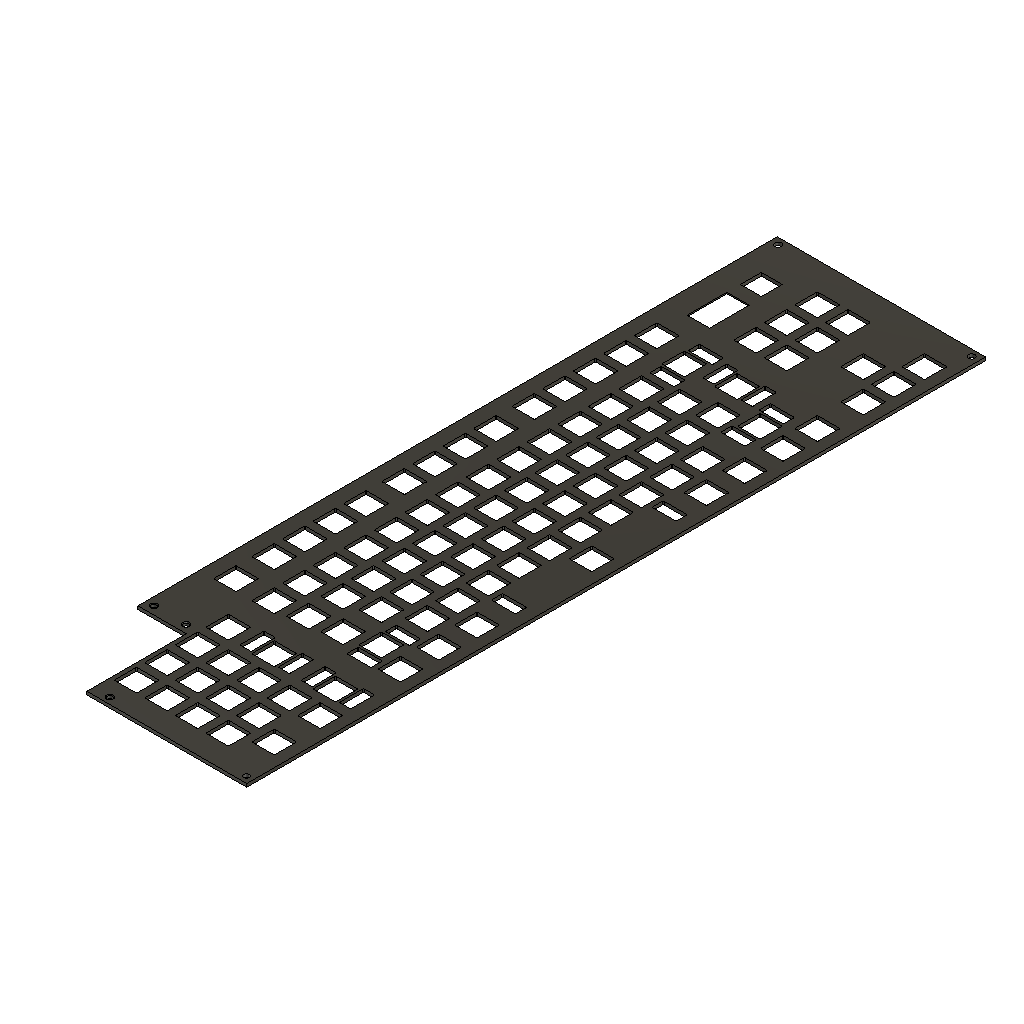
PCBPlate (Autodesk Fusion 360 design; units mm, degrees)
part number: 2026-06-08-16-43-16-633
Autodesk Fusion 360 part; units mm, degrees
(part 1 of 4)
sketch "IronHandPCBPlate" plane through (0, 0, 0) normal (0, 0, 1) x (1, 0, 0)
  arc A0 (-58.5792, -128.4193) -> (-59.0792, -127.9193) centre (-58.5792, -127.9193) cw
  arc A1 (-45.5792, -114.4193) -> (-45.0793, -114.9193) centre (-45.5793, -114.9193) cw
  line L0 (-45.0793, -114.9193) -> (-45.0793, -127.9193)
  line L1 (-59.0792, -127.9193) -> (-59.0793, -114.9193)
  arc A2 (-45.0793, -127.9193) -> (-45.5792, -128.4193) centre (-45.5792, -127.9193) cw
  line L2 (-58.5792, -114.4193) -> (-45.5792, -114.4193)
  line L3 (-45.5792, -128.4193) -> (-58.5792, -128.4193)
  arc A3 (-59.0793, -114.9193) -> (-58.5792, -114.4193) centre (-58.5793, -114.9193) cw
  line L4 (-59.0792, -104.1068) -> (-59.0792, -91.1068)
  line L5 (-45.5792, -104.6068) -> (-58.5792, -104.6068)
  arc A4 (-58.5792, -104.6068) -> (-59.0792, -104.1068) centre (-58.5792, -104.1068) cw
  arc A5 (-45.5793, -90.6068) -> (-45.0792, -91.1068) centre (-45.5792, -91.1068) cw
  arc A6 (-45.0792, -104.1068) -> (-45.5792, -104.6068) centre (-45.5792, -104.1068) cw
  arc A7 (-59.0792, -91.1068) -> (-58.5793, -90.6068) centre (-58.5792, -91.1068) cw
  line L6 (-58.5793, -90.6068) -> (-45.5793, -90.6068)
  line L7 (-45.0792, -91.1068) -> (-45.0792, -104.1068)
  line L8 (-58.5792, -71.5568) -> (-45.5792, -71.5568)
  arc A8 (-45.5792, -71.5568) -> (-45.0792, -72.0568) centre (-45.5792, -72.0568) cw
  line L9 (-45.0792, -72.0568) -> (-45.0792, -85.0568)
  arc A9 (-45.0792, -85.0568) -> (-45.5792, -85.5568) centre (-45.5792, -85.0568) cw
  line L10 (-59.0792, -85.0568) -> (-59.0792, -72.0568)
  line L11 (-45.5792, -85.5568) -> (-58.5792, -85.5568)
  arc A10 (-59.0792, -72.0568) -> (-58.5792, -71.5568) centre (-58.5792, -72.0568) cw
  arc A11 (-58.5792, -85.5568) -> (-59.0792, -85.0568) centre (-58.5792, -85.0568) cw
  arc A12 (-59.0793, -53.0068) -> (-58.5792, -52.5068) centre (-58.5792, -53.0068) cw
  line L12 (-58.5792, -52.5068) -> (-45.5792, -52.5068)
  arc A13 (-58.5792, -66.5068) -> (-59.0792, -66.0068) centre (-58.5792, -66.0068) cw
  line L13 (-45.0792, -53.0068) -> (-45.0793, -66.0068)
  line L14 (-59.0792, -66.0068) -> (-59.0793, -53.0068)
  arc A14 (-45.0793, -66.0068) -> (-45.5792, -66.5068) centre (-45.5792, -66.0068) cw
  arc A15 (-45.5792, -52.5068) -> (-45.0792, -53.0068) centre (-45.5792, -53.0068) cw
  line L15 (-45.5792, -66.5068) -> (-58.5792, -66.5068)
  line L16 (-45.0792, -33.9568) -> (-45.0792, -46.9568)
  line L17 (-58.5792, -33.4568) -> (-45.5792, -33.4568)
  arc A16 (-45.5792, -33.4568) -> (-45.0792, -33.9568) centre (-45.5792, -33.9568) cw
  arc A17 (-45.0792, -46.9568) -> (-45.5792, -47.4568) centre (-45.5792, -46.9568) cw
  arc A18 (-58.5792, -47.4568) -> (-59.0792, -46.9568) centre (-58.5792, -46.9568) cw
  line L18 (-45.5792, -47.4568) -> (-58.5792, -47.4568)
  line L19 (-59.0792, -46.9568) -> (-59.0793, -33.9568)
  arc A19 (-59.0793, -33.9568) -> (-58.5792, -33.4568) centre (-58.5792, -33.9568) cw
  line L20 (-58.5792, -9.6443) -> (-45.5792, -9.6443)
  line L21 (-45.5792, -23.6443) -> (-58.5792, -23.6443)
  arc A20 (-58.5792, -23.6443) -> (-59.0792, -23.1443) centre (-58.5792, -23.1443) cw
  line L22 (-45.0792, -10.1443) -> (-45.0793, -23.1443)
  arc A21 (-59.0793, -10.1443) -> (-58.5792, -9.6443) centre (-58.5792, -10.1443) cw
  arc A22 (-45.0793, -23.1443) -> (-45.5792, -23.6443) centre (-45.5792, -23.1443) cw
  line L23 (-59.0792, -23.1443) -> (-59.0793, -10.1443)
  arc A23 (-45.5792, -9.6443) -> (-45.0792, -10.1443) centre (-45.5792, -10.1443) cw
  line L24 (-45.5792, -4.5943) -> (-58.5792, -4.5943)
  line L25 (-59.0792, -4.0943) -> (-59.0793, 8.9057)
  line L26 (-45.0792, 8.9057) -> (-45.0792, -4.0943)
  arc A24 (-59.0793, 8.9057) -> (-58.5792, 9.4057) centre (-58.5792, 8.9057) cw
  arc A25 (-45.0792, -4.0943) -> (-45.5792, -4.5943) centre (-45.5792, -4.0943) cw
  arc A26 (-58.5792, -4.5943) -> (-59.0792, -4.0943) centre (-58.5792, -4.0943) cw
  line L27 (-58.5792, 9.4057) -> (-45.5792, 9.4057)
  arc A27 (-45.5792, 9.4057) -> (-45.0792, 8.9057) centre (-45.5792, 8.9057) cw
  line L28 (-59.0792, 14.9557) -> (-59.0792, 27.9557)
  line L29 (-45.5792, 14.4557) -> (-58.5792, 14.4557)
  line L30 (-58.5792, 28.4557) -> (-45.5792, 28.4557)
  arc A28 (-45.5792, 28.4557) -> (-45.0792, 27.9557) centre (-45.5792, 27.9557) cw
  arc A29 (-45.0792, 14.9557) -> (-45.5792, 14.4557) centre (-45.5792, 14.9557) cw
  line L31 (-45.0792, 27.9557) -> (-45.0792, 14.9557)
  arc A30 (-59.0792, 27.9557) -> (-58.5792, 28.4557) centre (-58.5792, 27.9557) cw
  arc A31 (-58.5792, 14.4557) -> (-59.0792, 14.9557) centre (-58.5793, 14.9557) cw
  line L32 (-45.5792, 33.5057) -> (-58.5792, 33.5057)
  line L33 (-58.5792, 47.5057) -> (-45.5792, 47.5057)
  line L34 (-45.0792, 47.0057) -> (-45.0792, 34.0057)
  arc A32 (-45.0792, 34.0057) -> (-45.5792, 33.5057) centre (-45.5792, 34.0057) cw
  arc A33 (-58.5792, 33.5057) -> (-59.0792, 34.0057) centre (-58.5792, 34.0057) cw
  line L35 (-59.0792, 34.0057) -> (-59.0793, 47.0057)
  arc A34 (-59.0793, 47.0057) -> (-58.5792, 47.5057) centre (-58.5792, 47.0057) cw
  arc A35 (-45.5792, 47.5057) -> (-45.0792, 47.0057) centre (-45.5792, 47.0057) cw
  arc A36 (-59.0793, 70.8182) -> (-58.5792, 71.3182) centre (-58.5792, 70.8182) cw
  line L36 (-59.0792, 57.8182) -> (-59.0793, 70.8182)
  arc A37 (-45.0792, 57.8182) -> (-45.5792, 57.3182) centre (-45.5792, 57.8182) cw
  line L37 (-45.0792, 70.8182) -> (-45.0792, 57.8182)
  arc A38 (-45.5792, 71.3182) -> (-45.0792, 70.8182) centre (-45.5792, 70.8182) cw
  arc A39 (-58.5792, 57.3182) -> (-59.0792, 57.8182) centre (-58.5792, 57.8182) cw
  line L38 (-45.5792, 57.3182) -> (-58.5792, 57.3182)
  line L39 (-58.5792, 71.3182) -> (-45.5792, 71.3182)
  line L40 (-59.0792, 76.8682) -> (-59.0792, 89.8682)
  arc A40 (-58.5792, 76.3682) -> (-59.0792, 76.8682) centre (-58.5792, 76.8682) cw
  line L41 (-58.5792, 90.3682) -> (-45.5792, 90.3682)
  line L42 (-45.5792, 76.3682) -> (-58.5792, 76.3682)
  arc A41 (-59.0792, 89.8682) -> (-58.5792, 90.3682) centre (-58.5792, 89.8682) cw
  line L43 (-45.0792, 89.8682) -> (-45.0792, 76.8682)
  arc A42 (-45.0792, 76.8682) -> (-45.5792, 76.3682) centre (-45.5792, 76.8682) cw
  arc A43 (-45.5792, 90.3682) -> (-45.0792, 89.8682) centre (-45.5792, 89.8682) cw
  line L44 (-59.0792, 95.9182) -> (-59.0792, 108.9182)
  line L45 (-45.5792, 95.4182) -> (-58.5792, 95.4182)
  arc A44 (-45.0792, 95.9182) -> (-45.5792, 95.4182) centre (-45.5792, 95.9182) cw
  arc A45 (-59.0792, 108.9182) -> (-58.5792, 109.4182) centre (-58.5792, 108.9182) cw
  line L46 (-45.0792, 108.9182) -> (-45.0792, 95.9182)
  arc A46 (-45.5792, 109.4182) -> (-45.0792, 108.9182) centre (-45.5792, 108.9182) cw
  arc A47 (-58.5792, 95.4182) -> (-59.0792, 95.9182) centre (-58.5792, 95.9182) cw
  line L47 (-58.5792, 109.4182) -> (-45.5792, 109.4182)
  line L48 (-58.5792, 128.4682) -> (-45.5792, 128.4682)
  line L49 (-45.5792, 114.4682) -> (-58.5792, 114.4682)
  arc A48 (-59.0792, 127.9682) -> (-58.5792, 128.4682) centre (-58.5792, 127.9682) cw
  line L50 (-45.0792, 127.9682) -> (-45.0792, 114.9682)
  arc A49 (-45.0792, 114.9682) -> (-45.5792, 114.4682) centre (-45.5792, 114.9682) cw
  line L51 (-59.0792, 114.9682) -> (-59.0792, 127.9682)
  arc A50 (-45.5792, 128.4682) -> (-45.0792, 127.9682) centre (-45.5792, 127.9682) cw
  arc A51 (-58.5792, 114.4682) -> (-59.0792, 114.9682) centre (-58.5792, 114.9682) cw
  line L52 (-58.5792, 147.5182) -> (-45.5792, 147.5182)
  line L53 (-59.0792, 134.0182) -> (-59.0793, 147.0182)
  arc A52 (-58.5792, 133.5182) -> (-59.0792, 134.0182) centre (-58.5792, 134.0182) cw
  arc A53 (-45.5792, 147.5182) -> (-45.0792, 147.0182) centre (-45.5792, 147.0182) cw
  line L54 (-45.0792, 147.0182) -> (-45.0792, 134.0182)
  arc A54 (-45.0792, 134.0182) -> (-45.5792, 133.5182) centre (-45.5792, 134.0182) cw
  arc A55 (-59.0793, 147.0182) -> (-58.5792, 147.5182) centre (-58.5792, 147.0182) cw
  line L55 (-45.5792, 133.5182) -> (-58.5792, 133.5182)
  arc A56 (-21.2667, -213.6443) -> (-21.7667, -214.1443) centre (-21.7668, -213.6443) cw
  arc A57 (-21.7667, -200.1443) -> (-21.2668, -200.6443) centre (-21.7667, -200.6443) cw
  line L56 (-21.2668, -200.6443) -> (-21.2667, -213.6443)
  arc A58 (-34.7667, -214.1443) -> (-35.2668, -213.6443) centre (-34.7667, -213.6443) cw
  line L57 (-35.2668, -213.6443) -> (-35.2667, -200.6443)
  line L58 (-21.7667, -214.1443) -> (-34.7667, -214.1443)
  line L59 (-34.7667, -200.1443) -> (-21.7667, -200.1443)
  arc A59 (-35.2667, -200.6443) -> (-34.7667, -200.1443) centre (-34.7667, -200.6443) cw
  line L60 (-34.7667, -181.0943) -> (-21.7667, -181.0943)
  arc A60 (-21.7667, -181.0943) -> (-21.2668, -181.5943) centre (-21.7668, -181.5943) cw
  arc A61 (-21.2667, -194.5943) -> (-21.7668, -195.0943) centre (-21.7667, -194.5943) cw
  arc A62 (-35.2668, -181.5943) -> (-34.7667, -181.0943) centre (-34.7667, -181.5943) cw
  line L61 (-21.2668, -181.5943) -> (-21.2667, -194.5943)
  line L62 (-21.7668, -195.0943) -> (-34.7668, -195.0943)
  arc A63 (-34.7668, -195.0943) -> (-35.2668, -194.5943) centre (-34.7667, -194.5943) cw
  line L63 (-35.2668, -194.5943) -> (-35.2668, -181.5943)
  arc A64 (-21.2667, -175.5443) -> (-21.7667, -176.0443) centre (-21.7667, -175.5443) cw
  arc A65 (-21.7667, -162.0443) -> (-21.2667, -162.5443) centre (-21.7667, -162.5443) cw
  arc A66 (-35.2667, -162.5443) -> (-34.7667, -162.0443) centre (-34.7667, -162.5443) cw
  line L64 (-35.2668, -175.5443) -> (-35.2667, -162.5443)
  line L65 (-34.7667, -162.0443) -> (-21.7667, -162.0443)
  arc A67 (-34.7667, -176.0443) -> (-35.2668, -175.5443) centre (-34.7667, -175.5443) cw
  line L66 (-21.7667, -176.0443) -> (-34.7667, -176.0443)
  line L67 (-21.2667, -162.5443) -> (-21.2667, -175.5443)
  arc A68 (-21.2667, -156.4943) -> (-21.7667, -156.9943) centre (-21.7667, -156.4943) cw
  line L68 (-35.2667, -156.4943) -> (-35.2667, -143.4943)
  line L69 (-21.7667, -156.9943) -> (-34.7667, -156.9943)
  arc A69 (-34.7667, -156.9943) -> (-35.2667, -156.4943) centre (-34.7667, -156.4943) cw
  line L70 (-21.2668, -143.4943) -> (-21.2667, -156.4943)
  arc A70 (-35.2667, -143.4943) -> (-34.7667, -142.9943) centre (-34.7667, -143.4943) cw
  line L71 (-34.7667, -142.9943) -> (-21.7667, -142.9943)
  arc A71 (-21.7667, -142.9943) -> (-21.2668, -143.4943) centre (-21.7667, -143.4943) cw
  arc A72 (-35.2668, -114.9193) -> (-34.7667, -114.4193) centre (-34.7668, -114.9193) cw
  line L72 (-35.2667, -127.9193) -> (-35.2668, -114.9193)
  arc A73 (-21.2667, -127.9193) -> (-21.7667, -128.4193) centre (-21.7667, -127.9193) cw
  arc A74 (-21.7667, -114.4193) -> (-21.2668, -114.9193) centre (-21.7667, -114.9193) cw
  arc A75 (-34.7667, -128.4193) -> (-35.2667, -127.9193) centre (-34.7667, -127.9193) cw
  line L73 (-21.7667, -128.4193) -> (-34.7667, -128.4193)
  line L74 (-34.7667, -114.4193) -> (-21.7667, -114.4193)
  line L75 (-21.2668, -114.9193) -> (-21.2667, -127.9193)
  arc A76 (-35.2667, -95.8693) -> (-34.7667, -95.3693) centre (-34.7667, -95.8693) cw
  arc A77 (-34.7667, -109.3693) -> (-35.2668, -108.8693) centre (-34.7667, -108.8693) cw
  arc A78 (-21.7667, -95.3693) -> (-21.2667, -95.8693) centre (-21.7667, -95.8693) cw
  line L76 (-21.2667, -95.8693) -> (-21.2668, -108.8693)
  arc A79 (-21.2667, -108.8693) -> (-21.7667, -109.3693) centre (-21.7667, -108.8693) cw
  line L77 (-35.2668, -108.8693) -> (-35.2667, -95.8693)
  line L78 (-21.7667, -109.3693) -> (-34.7667, -109.3693)
  line L79 (-34.7667, -95.3693) -> (-21.7667, -95.3693)
  line L80 (-21.7667, -90.3193) -> (-34.7667, -90.3193)
  arc A80 (-34.7667, -90.3193) -> (-35.2667, -89.8193) centre (-34.7667, -89.8193) cw
  line L81 (-21.2667, -76.8193) -> (-21.2667, -89.8193)
  line L82 (-34.7667, -76.3193) -> (-21.7667, -76.3193)
  arc A81 (-21.7667, -76.3193) -> (-21.2667, -76.8193) centre (-21.7667, -76.8193) cw
  line L83 (-35.2667, -89.8193) -> (-35.2667, -76.8193)
  arc A82 (-21.2667, -89.8193) -> (-21.7667, -90.3193) centre (-21.7667, -89.8193) cw
  arc A83 (-35.2667, -76.8193) -> (-34.7667, -76.3193) centre (-34.7667, -76.8193) cw
  line L84 (-21.7667, -71.2693) -> (-34.7667, -71.2693)
  arc A84 (-21.2667, -70.7693) -> (-21.7667, -71.2693) centre (-21.7667, -70.7693) cw
  line L85 (-21.2667, -57.7693) -> (-21.2667, -70.7693)
  arc A85 (-34.7667, -71.2693) -> (-35.2667, -70.7693) centre (-34.7667, -70.7693) cw
  arc A86 (-35.2667, -57.7693) -> (-34.7667, -57.2693) centre (-34.7667, -57.7693) cw
  line L86 (-34.7667, -57.2693) -> (-21.7667, -57.2693)
  line L87 (-35.2667, -70.7693) -> (-35.2667, -57.7693)
  arc A87 (-21.7667, -57.2693) -> (-21.2667, -57.7693) centre (-21.7667, -57.7693) cw
  line L88 (-21.7667, -52.2193) -> (-34.7667, -52.2193)
  line L89 (-34.7667, -38.2193) -> (-21.7667, -38.2193)
  arc A88 (-34.7667, -52.2193) -> (-35.2667, -51.7193) centre (-34.7667, -51.7193) cw
  arc A89 (-21.2667, -51.7193) -> (-21.7667, -52.2193) centre (-21.7667, -51.7193) cw
  line L90 (-21.2667, -38.7193) -> (-21.2667, -51.7193)
  arc A90 (-35.2667, -38.7193) -> (-34.7667, -38.2193) centre (-34.7667, -38.7193) cw
  arc A91 (-21.7667, -38.2193) -> (-21.2667, -38.7193) centre (-21.7667, -38.7193) cw
  line L91 (-35.2667, -51.7193) -> (-35.2667, -38.7193)
  arc A92 (-21.2667, -32.6693) -> (-21.7667, -33.1693) centre (-21.7667, -32.6693) cw
  arc A93 (-21.7667, -19.1693) -> (-21.2667, -19.6693) centre (-21.7667, -19.6693) cw
  line L92 (-34.7667, -19.1693) -> (-21.7667, -19.1693)
  line L93 (-21.2667, -19.6693) -> (-21.2667, -32.6693)
  arc A94 (-34.7667, -33.1693) -> (-35.2667, -32.6693) centre (-34.7667, -32.6693) cw
  line L94 (-21.7667, -33.1693) -> (-34.7667, -33.1693)
  line L95 (-35.2667, -32.6693) -> (-35.2667, -19.6693)
  arc A95 (-35.2667, -19.6693) -> (-34.7667, -19.1693) centre (-34.7667, -19.6693) cw
  arc A96 (-21.2667, -13.6193) -> (-21.7667, -14.1193) centre (-21.7667, -13.6193) cw
  line L96 (-21.2667, -0.6193) -> (-21.2667, -13.6193)
  arc A97 (-34.7667, -14.1193) -> (-35.2667, -13.6193) centre (-34.7667, -13.6193) cw
  line L97 (-35.2667, -13.6193) -> (-35.2667, -0.6193)
  arc A98 (-35.2667, -0.6193) -> (-34.7667, -0.1193) centre (-34.7667, -0.6193) cw
  line L98 (-21.7667, -14.1193) -> (-34.7667, -14.1193)
  arc A99 (-21.7667, -0.1193) -> (-21.2667, -0.6193) centre (-21.7667, -0.6193) cw
  line L99 (-34.7667, -0.1193) -> (-21.7667, -0.1193)
  line L100 (-21.7667, 4.9307) -> (-34.7667, 4.9307)
  arc A100 (-21.7667, 18.9307) -> (-21.2667, 18.4307) centre (-21.7667, 18.4307) cw
  arc A101 (-35.2667, 18.4307) -> (-34.7667, 18.9307) centre (-34.7667, 18.4307) cw
  line L101 (-35.2667, 5.4307) -> (-35.2667, 18.4307)
  line L102 (-21.2667, 18.4307) -> (-21.2667, 5.4307)
  arc A102 (-21.2667, 5.4307) -> (-21.7667, 4.9307) centre (-21.7667, 5.4307) cw
  line L103 (-34.7667, 18.9307) -> (-21.7667, 18.9307)
  arc A103 (-34.7667, 4.9307) -> (-35.2667, 5.4307) centre (-34.7667, 5.4307) cw
  arc A104 (-21.2667, 24.4807) -> (-21.7667, 23.9807) centre (-21.7667, 24.4807) cw
  arc A105 (-21.7667, 37.9807) -> (-21.2667, 37.4807) centre (-21.7667, 37.4807) cw
  arc A106 (-35.2667, 37.4807) -> (-34.7667, 37.9807) centre (-34.7667, 37.4807) cw
  line L104 (-35.2667, 24.4807) -> (-35.2667, 37.4807)
  line L105 (-21.2667, 37.4807) -> (-21.2667, 24.4807)
  arc A107 (-34.7667, 23.9807) -> (-35.2667, 24.4807) centre (-34.7667, 24.4807) cw
  line L106 (-34.7667, 37.9807) -> (-21.7667, 37.9807)
  line L107 (-21.7667, 23.9807) -> (-34.7667, 23.9807)
  line L108 (-21.2667, 56.5307) -> (-21.2667, 43.5307)
  line L109 (-35.2667, 43.5307) -> (-35.2667, 56.5307)
  arc A108 (-35.2667, 56.5307) -> (-34.7667, 57.0307) centre (-34.7667, 56.5307) cw
  line L110 (-34.7667, 57.0307) -> (-21.7667, 57.0307)
  arc A109 (-21.2667, 43.5307) -> (-21.7667, 43.0307) centre (-21.7667, 43.5307) cw
  arc A110 (-21.7667, 57.0307) -> (-21.2667, 56.5307) centre (-21.7667, 56.5307) cw
  line L111 (-21.7667, 43.0307) -> (-34.7667, 43.0307)
  arc A111 (-34.7667, 43.0307) -> (-35.2667, 43.5307) centre (-34.7667, 43.5307) cw
  arc A112 (-21.2667, 62.5807) -> (-21.7667, 62.0807) centre (-21.7667, 62.5807) cw
  line L112 (-34.7667, 76.0807) -> (-21.7667, 76.0807)
  line L113 (-21.7667, 62.0807) -> (-34.7667, 62.0807)
  arc A113 (-35.2667, 75.5807) -> (-34.7667, 76.0807) centre (-34.7667, 75.5807) cw
  arc A114 (-34.7667, 62.0807) -> (-35.2667, 62.5807) centre (-34.7667, 62.5807) cw
  line L114 (-21.2667, 75.5807) -> (-21.2667, 62.5807)
  arc A115 (-21.7667, 76.0807) -> (-21.2667, 75.5807) centre (-21.7667, 75.5807) cw
  line L115 (-35.2667, 62.5807) -> (-35.2667, 75.5807)
  arc A116 (-21.2667, 81.6307) -> (-21.7667, 81.1307) centre (-21.7667, 81.6307) cw
  arc A117 (-34.7667, 81.1307) -> (-35.2667, 81.6307) centre (-34.7667, 81.6307) cw
  line L116 (-34.7667, 95.1307) -> (-21.7667, 95.1307)
  arc A118 (-35.2667, 94.6307) -> (-34.7667, 95.1307) centre (-34.7667, 94.6307) cw
  arc A119 (-21.7667, 95.1307) -> (-21.2667, 94.6307) centre (-21.7667, 94.6307) cw
  line L117 (-21.7667, 81.1307) -> (-34.7667, 81.1307)
  line L118 (-21.2667, 94.6307) -> (-21.2667, 81.6307)
  line L119 (-35.2667, 81.6307) -> (-35.2667, 94.6307)
  line L120 (-35.2667, 100.6807) -> (-35.2667, 113.6807)
  line L121 (-21.2667, 113.6807) -> (-21.2667, 100.6807)
  line L122 (-34.7667, 114.1807) -> (-21.7667, 114.1807)
  line L123 (-21.7667, 100.1807) -> (-34.7667, 100.1807)
  arc A120 (-21.2667, 100.6807) -> (-21.7667, 100.1807) centre (-21.7667, 100.6807) cw
  arc A121 (-21.7667, 114.1807) -> (-21.2667, 113.6807) centre (-21.7667, 113.6807) cw
  arc A122 (-34.7667, 100.1807) -> (-35.2667, 100.6807) centre (-34.7667, 100.6807) cw
  arc A123 (-35.2667, 113.6807) -> (-34.7667, 114.1807) centre (-34.7667, 113.6807) cw
  line L124 (-34.7667, 140.8495) -> (-21.7667, 140.8495)
  line L125 (-21.2667, 140.3495) -> (-21.2667, 127.3495)
  arc A124 (-21.2667, 127.3495) -> (-21.7667, 126.8495) centre (-21.7667, 127.3495) cw
  arc A125 (-34.7667, 126.8495) -> (-35.2667, 127.3495) centre (-34.7667, 127.3495) cw
  line L126 (-35.2667, 127.3495) -> (-35.2667, 140.3495)
  arc A126 (-21.7667, 140.8495) -> (-21.2667, 140.3495) centre (-21.7667, 140.3495) cw
  line L127 (-21.7667, 126.8495) -> (-34.7667, 126.8495)
  arc A127 (-35.2667, 140.3495) -> (-34.7667, 140.8495) centre (-34.7667, 140.3495) cw
  line L128 (-25.7417, 162.5932) -> (-25.7417, 175.5932)
  arc A128 (-12.2417, 176.0932) -> (-11.7417, 175.5932) centre (-12.2417, 175.5932) cw
  line L129 (-25.2417, 176.0932) -> (-12.2417, 176.0932)
  line L130 (-11.7417, 175.5932) -> (-11.7417, 162.5932)
  line L131 (-12.2417, 162.0932) -> (-25.2417, 162.0932)
  arc A129 (-11.7417, 162.5932) -> (-12.2417, 162.0932) centre (-12.2417, 162.5932) cw
  arc A130 (-25.7417, 175.5932) -> (-25.2417, 176.0932) centre (-25.2417, 175.5932) cw
  arc A131 (-25.2417, 162.0932) -> (-25.7417, 162.5932) centre (-25.2417, 162.5932) cw
  arc A132 (-25.7417, 194.6432) -> (-25.2417, 195.1432) centre (-25.2417, 194.6432) cw
  line L132 (-12.2417, 181.1432) -> (-25.2417, 181.1432)
  arc A133 (-11.7417, 181.6432) -> (-12.2417, 181.1432) centre (-12.2417, 181.6432) cw
  line L133 (-11.7417, 194.6432) -> (-11.7417, 181.6432)
  line L134 (-25.2417, 195.1432) -> (-12.2417, 195.1432)
  arc A134 (-25.2417, 181.1432) -> (-25.7417, 181.6432) centre (-25.2417, 181.6432) cw
  line L135 (-25.7417, 181.6432) -> (-25.7417, 194.6432)
  arc A135 (-12.2417, 195.1432) -> (-11.7417, 194.6432) centre (-12.2417, 194.6432) cw
  arc A136 (-11.7417, 200.6932) -> (-12.2417, 200.1932) centre (-12.2417, 200.6932) cw
  line L136 (-25.2417, 214.1932) -> (-12.2417, 214.1932)
  line L137 (-11.7417, 213.6932) -> (-11.7417, 200.6932)
  line L138 (-12.2417, 200.1932) -> (-25.2417, 200.1932)
  arc A137 (-25.7417, 213.6932) -> (-25.2417, 214.1932) centre (-25.2417, 213.6932) cw
  line L139 (-25.7417, 200.6932) -> (-25.7417, 213.6932)
  arc A138 (-25.2417, 200.1932) -> (-25.7417, 200.6932) centre (-25.2417, 200.6932) cw
  arc A139 (-12.2417, 214.1932) -> (-11.7417, 213.6932) centre (-12.2417, 213.6932) cw
  line L140 (-2.7168, -214.1443) -> (-15.7168, -214.1443)
  line L141 (-16.2168, -213.6443) -> (-16.2168, -200.6443)
  arc A140 (-2.2168, -213.6443) -> (-2.7168, -214.1443) centre (-2.7168, -213.6443) cw
  line L142 (-15.7167, -200.1443) -> (-2.7168, -200.1443)
  arc A141 (-2.7168, -200.1443) -> (-2.2167, -200.6443) centre (-2.7167, -200.6443) cw
  line L143 (-2.2167, -200.6443) -> (-2.2168, -213.6443)
  arc A142 (-15.7168, -214.1443) -> (-16.2168, -213.6443) centre (-15.7167, -213.6443) cw
  arc A143 (-16.2168, -200.6443) -> (-15.7167, -200.1443) centre (-15.7168, -200.6443) cw
  arc A144 (-15.7168, -195.0943) -> (-16.2167, -194.5943) centre (-15.7167, -194.5943) cw
  line L144 (-16.2167, -194.5943) -> (-16.2168, -181.5943)
  line L145 (-2.2167, -181.5943) -> (-2.2167, -194.5943)
  line L146 (-15.7167, -181.0943) -> (-2.7168, -181.0943)
  line L147 (-2.7168, -195.0943) -> (-15.7168, -195.0943)
  arc A145 (-2.7168, -181.0943) -> (-2.2168, -181.5943) centre (-2.7167, -181.5943) cw
  arc A146 (-2.2167, -194.5943) -> (-2.7168, -195.0943) centre (-2.7167, -194.5943) cw
  arc A147 (-16.2168, -181.5943) -> (-15.7167, -181.0943) centre (-15.7167, -181.5943) cw
  arc A148 (-2.2168, -175.5443) -> (-2.7168, -176.0443) centre (-2.7167, -175.5443) cw
  arc A149 (-15.7167, -176.0443) -> (-16.2168, -175.5443) centre (-15.7168, -175.5443) cw
  arc A150 (-16.2168, -162.5443) -> (-15.7167, -162.0443) centre (-15.7167, -162.5443) cw
  line L148 (-16.2168, -175.5443) -> (-16.2168, -162.5443)
  arc A151 (-2.7168, -162.0443) -> (-2.2167, -162.5443) centre (-2.7168, -162.5443) cw
  line L149 (-2.2167, -162.5443) -> (-2.2168, -175.5443)
  line L150 (-2.7168, -176.0443) -> (-15.7167, -176.0443)
  line L151 (-15.7167, -162.0443) -> (-2.7168, -162.0443)
  arc A152 (7.3082, -156.4943) -> (6.8083, -156.9943) centre (6.8082, -156.4943) cw
  line L152 (-6.1917, -142.9943) -> (6.8083, -142.9943)
  arc A153 (-6.6917, -143.4943) -> (-6.1917, -142.9943) centre (-6.1917, -143.4943) cw
  line L153 (7.3082, -143.4943) -> (7.3082, -156.4943)
  arc A154 (6.8083, -142.9943) -> (7.3082, -143.4943) centre (6.8083, -143.4943) cw
  line L154 (-6.6917, -156.4943) -> (-6.6917, -143.4943)
  line L155 (6.8083, -156.9943) -> (-6.1917, -156.9943)
  arc A155 (-6.1917, -156.9943) -> (-6.6917, -156.4943) centre (-6.1918, -156.4943) cw
  line L156 (-15.1297, -155.4943) -> (-15.1297, -141.4943)
  arc A156 (-8.6297, -140.9943) -> (-8.1297, -141.4943) centre (-8.6297, -141.4943) cw
  line L157 (-14.6298, -140.9943) -> (-8.6297, -140.9943)
  line L158 (-8.6297, -155.9943) -> (-14.6298, -155.9943)
  arc A157 (-15.1297, -141.4943) -> (-14.6298, -140.9943) centre (-14.6297, -141.4943) cw
  arc A158 (-14.6298, -155.9943) -> (-15.1297, -155.4943) centre (-14.6297, -155.4943) cw
  arc A159 (-8.1297, -155.4943) -> (-8.6297, -155.9943) centre (-8.6297, -155.4943) cw
  line L159 (-8.1297, -141.4943) -> (-8.1297, -155.4943)
  arc A160 (9.2463, -155.9943) -> (8.7463, -155.4943) centre (9.2462, -155.4943) cw
  line L160 (8.7463, -155.4943) -> (8.7463, -141.4943)
  line L161 (15.2463, -155.9943) -> (9.2463, -155.9943)
  line L162 (15.7463, -141.4943) -> (15.7463, -155.4943)
  arc A161 (15.2463, -140.9943) -> (15.7463, -141.4943) centre (15.2463, -141.4943) cw
  arc A162 (8.7463, -141.4943) -> (9.2463, -140.9943) centre (9.2463, -141.4943) cw
  line L163 (9.2463, -140.9943) -> (15.2463, -140.9943)
  arc A163 (15.7463, -155.4943) -> (15.2463, -155.9943) centre (15.2463, -155.4943) cw
  arc A164 (-2.2167, -125.538) -> (-2.7167, -126.038) centre (-2.7167, -125.538) cw
  line L164 (-2.7167, -126.038) -> (-15.7167, -126.038)
  line L165 (-2.2167, -112.538) -> (-2.2167, -125.538)
  line L166 (-15.7167, -112.038) -> (-2.7167, -112.038)
  arc A165 (-2.7167, -112.038) -> (-2.2167, -112.538) centre (-2.7167, -112.538) cw
  line L167 (-16.2168, -125.538) -> (-16.2167, -112.538)
  arc A166 (-16.2167, -112.538) -> (-15.7167, -112.038) centre (-15.7167, -112.538) cw
  arc A167 (-15.7167, -126.038) -> (-16.2168, -125.538) centre (-15.7167, -125.538) cw
  line L168 (-2.2167, -91.1068) -> (-2.2167, -104.1068)
  arc A168 (-2.2167, -104.1068) -> (-2.7167, -104.6068) centre (-2.7167, -104.1068) cw
  line L169 (-16.2167, -104.1068) -> (-16.2167, -91.1068)
  arc A169 (-16.2167, -91.1068) -> (-15.7167, -90.6068) centre (-15.7167, -91.1068) cw
  line L170 (-2.7167, -104.6068) -> (-15.7167, -104.6068)
  arc A170 (-15.7167, -104.6068) -> (-16.2167, -104.1068) centre (-15.7167, -104.1068) cw
  arc A171 (-2.7167, -90.6068) -> (-2.2167, -91.1068) centre (-2.7167, -91.1068) cw
  line L171 (-15.7167, -90.6068) -> (-2.7167, -90.6068)
  line L172 (-2.2167, -72.0568) -> (-2.2167, -85.0568)
  arc A172 (-15.7167, -85.5568) -> (-16.2167, -85.0568) centre (-15.7167, -85.0568) cw
  line L173 (-16.2167, -85.0568) -> (-16.2167, -72.0568)
  arc A173 (-2.7167, -71.5568) -> (-2.2167, -72.0568) centre (-2.7167, -72.0568) cw
  arc A174 (-16.2167, -72.0568) -> (-15.7167, -71.5568) centre (-15.7167, -72.0568) cw
  line L174 (-15.7167, -71.5568) -> (-2.7167, -71.5568)
  arc A175 (-2.2167, -85.0568) -> (-2.7167, -85.5568) centre (-2.7167, -85.0568) cw
  line L175 (-2.7167, -85.5568) -> (-15.7167, -85.5568)
  arc A176 (-15.7167, -66.5068) -> (-16.2167, -66.0068) centre (-15.7167, -66.0068) cw
  line L176 (-2.7167, -66.5068) -> (-15.7167, -66.5068)
  arc A177 (-2.2167, -66.0068) -> (-2.7167, -66.5068) centre (-2.7167, -66.0068) cw
  arc A178 (-2.7167, -52.5068) -> (-2.2167, -53.0068) centre (-2.7167, -53.0068) cw
  line L177 (-2.2167, -53.0068) -> (-2.2167, -66.0068)
  arc A179 (-16.2167, -53.0068) -> (-15.7167, -52.5068) centre (-15.7167, -53.0068) cw
  line L178 (-16.2167, -66.0068) -> (-16.2167, -53.0068)
  line L179 (-15.7167, -52.5068) -> (-2.7167, -52.5068)
  arc A180 (-16.2167, -33.9568) -> (-15.7167, -33.4568) centre (-15.7167, -33.9568) cw
  line L180 (-2.2167, -33.9568) -> (-2.2167, -46.9568)
  line L181 (-16.2167, -46.9568) -> (-16.2167, -33.9568)
  line L182 (-2.7167, -47.4568) -> (-15.7167, -47.4568)
  arc A181 (-2.2167, -46.9568) -> (-2.7167, -47.4568) centre (-2.7167, -46.9568) cw
  arc A182 (-2.7167, -33.4568) -> (-2.2167, -33.9568) centre (-2.7167, -33.9568) cw
  arc A183 (-15.7167, -47.4568) -> (-16.2167, -46.9568) centre (-15.7167, -46.9568) cw
  line L183 (-15.7167, -33.4568) -> (-2.7167, -33.4568)
  arc A184 (-16.2167, -14.9068) -> (-15.7167, -14.4068) centre (-15.7167, -14.9068) cw
  line L184 (-16.2167, -27.9068) -> (-16.2167, -14.9068)
  line L185 (-2.7167, -28.4068) -> (-15.7167, -28.4068)
  arc A185 (-2.2167, -27.9068) -> (-2.7167, -28.4068) centre (-2.7167, -27.9068) cw
  line L186 (-15.7167, -14.4068) -> (-2.7167, -14.4068)
  arc A186 (-15.7167, -28.4068) -> (-16.2167, -27.9068) centre (-15.7167, -27.9068) cw
  line L187 (-2.2167, -14.9068) -> (-2.2167, -27.9068)
  arc A187 (-2.7167, -14.4068) -> (-2.2167, -14.9068) centre (-2.7167, -14.9068) cw
  arc A188 (-16.2167, 4.1432) -> (-15.7167, 4.6432) centre (-15.7167, 4.1432) cw
  line L188 (-2.2167, 4.1432) -> (-2.2167, -8.8568)
  line L189 (-2.7167, -9.3568) -> (-15.7167, -9.3568)
  line L190 (-16.2167, -8.8568) -> (-16.2167, 4.1432)
  arc A189 (-2.7167, 4.6432) -> (-2.2167, 4.1432) centre (-2.7167, 4.1432) cw
  arc A190 (-2.2167, -8.8568) -> (-2.7167, -9.3568) centre (-2.7167, -8.8568) cw
  arc A191 (-15.7167, -9.3568) -> (-16.2167, -8.8568) centre (-15.7167, -8.8568) cw
  line L191 (-15.7167, 4.6432) -> (-2.7167, 4.6432)
  arc A192 (-2.7167, 23.6932) -> (-2.2167, 23.1932) centre (-2.7167, 23.1932) cw
  arc A193 (-15.7167, 9.6932) -> (-16.2167, 10.1932) centre (-15.7167, 10.1932) cw
  line L192 (-2.2167, 23.1932) -> (-2.2167, 10.1932)
  line L193 (-16.2167, 10.1932) -> (-16.2167, 23.1932)
  arc A194 (-2.2167, 10.1932) -> (-2.7167, 9.6932) centre (-2.7167, 10.1932) cw
  arc A195 (-16.2167, 23.1932) -> (-15.7167, 23.6932) centre (-15.7167, 23.1932) cw
  line L194 (-15.7167, 23.6932) -> (-2.7167, 23.6932)
  line L195 (-2.7167, 9.6932) -> (-15.7167, 9.6932)
  arc A196 (-2.7167, 42.7432) -> (-2.2167, 42.2432) centre (-2.7167, 42.2432) cw
  line L196 (-2.7167, 28.7432) -> (-15.7167, 28.7432)
  line L197 (-15.7167, 42.7432) -> (-2.7167, 42.7432)
  line L198 (-2.2167, 42.2432) -> (-2.2167, 29.2432)
  arc A197 (-2.2167, 29.2432) -> (-2.7167, 28.7432) centre (-2.7167, 29.2432) cw
  arc A198 (-15.7167, 28.7432) -> (-16.2167, 29.2432) centre (-15.7167, 29.2432) cw
  line L199 (-16.2167, 29.2432) -> (-16.2167, 42.2432)
  arc A199 (-16.2167, 42.2432) -> (-15.7167, 42.7432) centre (-15.7167, 42.2432) cw
  line L200 (-16.2167, 48.2932) -> (-16.2167, 61.2932)
  line L201 (-2.7167, 47.7932) -> (-15.7167, 47.7932)
  arc A200 (-2.7167, 61.7932) -> (-2.2167, 61.2932) centre (-2.7167, 61.2932) cw
  line L202 (-2.2167, 61.2932) -> (-2.2167, 48.2932)
  arc A201 (-16.2167, 61.2932) -> (-15.7167, 61.7932) centre (-15.7167, 61.2932) cw
  arc A202 (-2.2167, 48.2932) -> (-2.7167, 47.7932) centre (-2.7167, 48.2932) cw
  arc A203 (-15.7167, 47.7932) -> (-16.2167, 48.2932) centre (-15.7167, 48.2932) cw
  line L203 (-15.7167, 61.7932) -> (-2.7167, 61.7932)
  arc A204 (-2.7167, 80.8432) -> (-2.2167, 80.3432) centre (-2.7167, 80.3432) cw
  line L204 (-16.2167, 67.3432) -> (-16.2167, 80.3432)
  line L205 (-2.2167, 80.3432) -> (-2.2167, 67.3432)
  arc A205 (-15.7167, 66.8432) -> (-16.2167, 67.3432) centre (-15.7167, 67.3432) cw
  line L206 (-2.7167, 66.8432) -> (-15.7167, 66.8432)
  line L207 (-15.7167, 80.8432) -> (-2.7167, 80.8432)
  arc A206 (-16.2167, 80.3432) -> (-15.7167, 80.8432) centre (-15.7167, 80.3432) cw
  arc A207 (-2.2167, 67.3432) -> (-2.7167, 66.8432) centre (-2.7167, 67.3432) cw
  line L208 (-15.7167, 99.8932) -> (-2.7167, 99.8932)
  arc A208 (-2.7167, 99.8932) -> (-2.2167, 99.3932) centre (-2.7167, 99.3932) cw
  arc A209 (-16.2167, 99.3932) -> (-15.7167, 99.8932) centre (-15.7167, 99.3932) cw
  arc A210 (-2.2167, 86.3932) -> (-2.7167, 85.8932) centre (-2.7167, 86.3932) cw
  line L209 (-2.7167, 85.8932) -> (-15.7167, 85.8932)
  line L210 (-2.2167, 99.3932) -> (-2.2167, 86.3932)
  line L211 (-16.2167, 86.3932) -> (-16.2167, 99.3932)
  arc A211 (-15.7167, 85.8932) -> (-16.2167, 86.3932) centre (-15.7167, 86.3932) cw
  line L212 (-16.2167, 105.4432) -> (-16.2167, 118.4432)
  arc A212 (-16.2167, 118.4432) -> (-15.7167, 118.9432) centre (-15.7167, 118.4432) cw
  arc A213 (-15.7167, 104.9432) -> (-16.2167, 105.4432) centre (-15.7167, 105.4432) cw
  line L213 (-2.7167, 104.9432) -> (-15.7167, 104.9432)
  arc A214 (-2.2167, 105.4432) -> (-2.7167, 104.9432) centre (-2.7167, 105.4432) cw
  arc A215 (-2.7167, 118.9432) -> (-2.2167, 118.4432) centre (-2.7167, 118.4432) cw
  line L214 (-2.2167, 118.4432) -> (-2.2167, 105.4432)
  line L215 (-15.7167, 118.9432) -> (-2.7167, 118.9432)
  line L216 (6.8083, 131.137) -> (-6.1917, 131.137)
  arc A216 (-6.6917, 144.637) -> (-6.1917, 145.137) centre (-6.1917, 144.637) cw
  arc A217 (6.8083, 145.137) -> (7.3083, 144.637) centre (6.8083, 144.637) cw
  line L217 (7.3083, 144.637) -> (7.3083, 131.637)
  arc A218 (-6.1917, 131.137) -> (-6.6917, 131.637) centre (-6.1917, 131.637) cw
  line L218 (-6.1917, 145.137) -> (6.8083, 145.137)
  arc A219 (7.3083, 131.637) -> (6.8083, 131.137) centre (6.8083, 131.637) cw
  line L219 (-6.6917, 131.637) -> (-6.6917, 144.637)
  arc A220 (-8.6297, 147.137) -> (-8.1297, 146.637) centre (-8.6297, 146.637) cw
  line L220 (-14.6297, 147.137) -> (-8.6297, 147.137)
  arc A221 (-14.6297, 132.137) -> (-15.1297, 132.637) centre (-14.6297, 132.637) cw
  line L221 (-15.1297, 132.637) -> (-15.1297, 146.637)
  arc A222 (-8.1297, 132.637) -> (-8.6297, 132.137) centre (-8.6297, 132.637) cw
  line L222 (-8.6297, 132.137) -> (-14.6297, 132.137)
  arc A223 (-15.1297, 146.637) -> (-14.6297, 147.137) centre (-14.6297, 146.637) cw
  line L223 (-8.1297, 146.637) -> (-8.1297, 132.637)
  line L224 (15.2463, 132.137) -> (9.2463, 132.137)
  line L225 (15.7463, 146.637) -> (15.7463, 132.637)
  line L226 (8.7463, 132.637) -> (8.7463, 146.637)
  arc A224 (9.2463, 132.137) -> (8.7463, 132.637) centre (9.2463, 132.637) cw
  arc A225 (15.7463, 132.637) -> (15.2463, 132.137) centre (15.2463, 132.637) cw
  arc A226 (8.7463, 146.637) -> (9.2463, 147.137) centre (9.2463, 146.637) cw
  arc A227 (15.2463, 147.137) -> (15.7463, 146.637) centre (15.2463, 146.637) cw
  line L227 (9.2463, 147.137) -> (15.2463, 147.137)
  line L228 (-6.1917, 176.0932) -> (6.8083, 176.0932)
  arc A228 (-6.1917, 162.0932) -> (-6.6917, 162.5932) centre (-6.1917, 162.5932) cw
  line L229 (6.8083, 162.0932) -> (-6.1917, 162.0932)
  arc A229 (-6.6917, 175.5932) -> (-6.1917, 176.0932) centre (-6.1917, 175.5932) cw
  line L230 (7.3083, 175.5932) -> (7.3083, 162.5932)
  arc A230 (6.8083, 176.0932) -> (7.3083, 175.5932) centre (6.8083, 175.5932) cw
  arc A231 (7.3083, 162.5932) -> (6.8083, 162.0932) centre (6.8083, 162.5932) cw
  line L231 (-6.6917, 162.5932) -> (-6.6917, 175.5932)
  arc A232 (-6.6917, 194.6432) -> (-6.1917, 195.1432) centre (-6.1917, 194.6432) cw
  line L232 (7.3083, 194.6432) -> (7.3083, 181.6432)
  arc A233 (7.3083, 181.6432) -> (6.8083, 181.1432) centre (6.8083, 181.6432) cw
  arc A234 (-6.1917, 181.1432) -> (-6.6917, 181.6432) centre (-6.1917, 181.6432) cw
  line L233 (-6.6917, 181.6432) -> (-6.6917, 194.6432)
  line L234 (6.8083, 181.1432) -> (-6.1917, 181.1432)
  arc A235 (6.8083, 195.1432) -> (7.3083, 194.6432) centre (6.8083, 194.6432) cw
  line L235 (-6.1917, 195.1432) -> (6.8083, 195.1432)
  arc A236 (6.8083, 214.1932) -> (7.3083, 213.6932) centre (6.8083, 213.6932) cw
  arc A237 (-6.6917, 213.6932) -> (-6.1917, 214.1932) centre (-6.1917, 213.6932) cw
  line L236 (-6.1917, 214.1932) -> (6.8083, 214.1932)
  line L237 (-6.6917, 200.6932) -> (-6.6917, 213.6932)
  line L238 (7.3083, 213.6932) -> (7.3083, 200.6932)
  line L239 (6.8083, 200.1932) -> (-6.1917, 200.1932)
  arc A238 (7.3083, 200.6932) -> (6.8083, 200.1932) centre (6.8083, 200.6932) cw
  arc A239 (-6.1917, 200.1932) -> (-6.6917, 200.6932) centre (-6.1917, 200.6932) cw
  line L240 (16.8333, -200.6443) -> (16.8332, -213.6443)
  arc A240 (2.8332, -200.6443) -> (3.3332, -200.1443) centre (3.3332, -200.6443) cw
  arc A241 (16.8332, -213.6443) -> (16.3333, -214.1443) centre (16.3332, -213.6443) cw
  line L241 (16.3333, -214.1443) -> (3.3332, -214.1443)
  arc A242 (3.3332, -214.1443) -> (2.8332, -213.6443) centre (3.3333, -213.6443) cw
  arc A243 (16.3333, -200.1443) -> (16.8333, -200.6443) centre (16.3333, -200.6443) cw
  line L242 (2.8332, -213.6443) -> (2.8332, -200.6443)
  line L243 (3.3332, -200.1443) -> (16.3333, -200.1443)
  arc A244 (3.3332, -195.0943) -> (2.8333, -194.5943) centre (3.3332, -194.5943) cw
  arc A245 (16.3333, -181.0943) -> (16.8333, -181.5943) centre (16.3333, -181.5943) cw
  line L244 (3.3332, -181.0943) -> (16.3333, -181.0943)
  line L245 (2.8333, -194.5943) -> (2.8332, -181.5943)
  arc A246 (16.8333, -194.5943) -> (16.3333, -195.0943) centre (16.3333, -194.5943) cw
  line L246 (16.3333, -195.0943) -> (3.3332, -195.0943)
  arc A247 (2.8332, -181.5943) -> (3.3332, -181.0943) centre (3.3333, -181.5943) cw
  line L247 (16.8333, -181.5943) -> (16.8333, -194.5943)
  arc A248 (16.8332, -175.5443) -> (16.3333, -176.0443) centre (16.3333, -175.5443) cw
  arc A249 (2.8332, -162.5443) -> (3.3332, -162.0443) centre (3.3333, -162.5443) cw
  line L248 (16.8333, -162.5443) -> (16.8332, -175.5443)
  line L249 (16.3333, -176.0443) -> (3.3332, -176.0443)
  line L250 (3.3332, -162.0443) -> (16.3333, -162.0443)
  arc A250 (16.3333, -162.0443) -> (16.8333, -162.5443) centre (16.3333, -162.5443) cw
  arc A251 (3.3332, -176.0443) -> (2.8333, -175.5443) centre (3.3332, -175.5443) cw
  line L251 (2.8333, -175.5443) -> (2.8332, -162.5443)
  line L252 (16.8333, -110.1568) -> (16.8333, -123.1568)
  line L253 (3.3333, -109.6568) -> (16.3333, -109.6568)
  arc A252 (3.3333, -123.6568) -> (2.8333, -123.1568) centre (3.3333, -123.1568) cw
  arc A253 (16.3333, -109.6568) -> (16.8333, -110.1568) centre (16.3333, -110.1568) cw
  arc A254 (16.8333, -123.1568) -> (16.3333, -123.6568) centre (16.3333, -123.1568) cw
  line L254 (16.3333, -123.6568) -> (3.3333, -123.6568)
  arc A255 (2.8333, -110.1568) -> (3.3333, -109.6568) centre (3.3333, -110.1568) cw
  line L255 (2.8333, -123.1568) -> (2.8333, -110.1568)
  line L256 (16.8333, -86.3443) -> (16.8333, -99.3443)
  arc A256 (3.3333, -99.8443) -> (2.8333, -99.3443) centre (3.3333, -99.3443) cw
  line L257 (16.3333, -99.8443) -> (3.3333, -99.8443)
  line L258 (3.3333, -85.8443) -> (16.3333, -85.8443)
  line L259 (2.8333, -99.3443) -> (2.8332, -86.3443)
  arc A257 (2.8332, -86.3443) -> (3.3333, -85.8443) centre (3.3333, -86.3443) cw
  arc A258 (16.8333, -99.3443) -> (16.3333, -99.8443) centre (16.3333, -99.3443) cw
  arc A259 (16.3333, -85.8443) -> (16.8333, -86.3443) centre (16.3333, -86.3443) cw
  arc A260 (16.8333, -80.2943) -> (16.3333, -80.7943) centre (16.3333, -80.2943) cw
  line L260 (16.3333, -80.7943) -> (3.3333, -80.7943)
  line L261 (2.8333, -80.2943) -> (2.8333, -67.2943)
  line L262 (3.3333, -66.7943) -> (16.3333, -66.7943)
  arc A261 (16.3333, -66.7943) -> (16.8333, -67.2943) centre (16.3333, -67.2943) cw
  arc A262 (3.3333, -80.7943) -> (2.8333, -80.2943) centre (3.3333, -80.2943) cw
  line L263 (16.8333, -67.2943) -> (16.8333, -80.2943)
  arc A263 (2.8333, -67.2943) -> (3.3333, -66.7943) centre (3.3333, -67.2943) cw
  line L264 (3.3333, -47.7443) -> (16.3333, -47.7443)
  arc A264 (16.8333, -61.2443) -> (16.3333, -61.7443) centre (16.3333, -61.2443) cw
  line L265 (2.8333, -61.2443) -> (2.8333, -48.2443)
  line L266 (16.3333, -61.7443) -> (3.3333, -61.7443)
  arc A265 (2.8333, -48.2443) -> (3.3333, -47.7443) centre (3.3333, -48.2443) cw
  line L267 (16.8333, -48.2443) -> (16.8333, -61.2443)
  arc A266 (3.3333, -61.7443) -> (2.8333, -61.2443) centre (3.3333, -61.2443) cw
  arc A267 (16.3333, -47.7443) -> (16.8333, -48.2443) centre (16.3333, -48.2443) cw
  line L268 (3.3333, -28.6943) -> (16.3333, -28.6943)
  arc A268 (16.8333, -42.1943) -> (16.3333, -42.6943) centre (16.3333, -42.1943) cw
  arc A269 (3.3333, -42.6943) -> (2.8333, -42.1943) centre (3.3333, -42.1943) cw
  arc A270 (2.8333, -29.1943) -> (3.3333, -28.6943) centre (3.3333, -29.1943) cw
  line L269 (2.8333, -42.1943) -> (2.8333, -29.1943)
  arc A271 (16.3333, -28.6943) -> (16.8333, -29.1943) centre (16.3333, -29.1943) cw
  line L270 (16.3333, -42.6943) -> (3.3333, -42.6943)
  line L271 (16.8333, -29.1943) -> (16.8333, -42.1943)
  line L272 (16.8333, -10.1443) -> (16.8333, -23.1443)
  arc A272 (3.3333, -23.6443) -> (2.8333, -23.1443) centre (3.3333, -23.1443) cw
  line L273 (2.8333, -23.1443) -> (2.8333, -10.1443)
  line L274 (3.3333, -9.6443) -> (16.3333, -9.6443)
  line L275 (16.3333, -23.6443) -> (3.3333, -23.6443)
  arc A273 (16.3333, -9.6443) -> (16.8333, -10.1443) centre (16.3333, -10.1443) cw
  arc A274 (2.8333, -10.1443) -> (3.3333, -9.6443) centre (3.3333, -10.1443) cw
  arc A275 (16.8333, -23.1443) -> (16.3333, -23.6443) centre (16.3333, -23.1443) cw
  line L276 (16.8333, 8.9057) -> (16.8333, -4.0943)
  line L277 (16.3333, -4.5943) -> (3.3333, -4.5943)
  arc A276 (16.8333, -4.0943) -> (16.3333, -4.5943) centre (16.3333, -4.0943) cw
  arc A277 (3.3333, -4.5943) -> (2.8333, -4.0943) centre (3.3333, -4.0943) cw
  arc A278 (16.3333, 9.4057) -> (16.8333, 8.9057) centre (16.3333, 8.9057) cw
  line L278 (2.8333, -4.0943) -> (2.8333, 8.9057)
  line L279 (3.3333, 9.4057) -> (16.3333, 9.4057)
  arc A279 (2.8333, 8.9057) -> (3.3333, 9.4057) centre (3.3333, 8.9057) cw
  arc A280 (2.8333, 27.9557) -> (3.3333, 28.4557) centre (3.3333, 27.9557) cw
  arc A281 (16.8333, 14.9557) -> (16.3333, 14.4557) centre (16.3333, 14.9557) cw
  arc A282 (3.3333, 14.4557) -> (2.8333, 14.9557) centre (3.3333, 14.9557) cw
  arc A283 (16.3333, 28.4557) -> (16.8333, 27.9557) centre (16.3333, 27.9557) cw
  line L280 (16.3333, 14.4557) -> (3.3333, 14.4557)
  line L281 (16.8333, 27.9557) -> (16.8333, 14.9557)
  line L282 (3.3333, 28.4557) -> (16.3333, 28.4557)
  line L283 (2.8333, 14.9557) -> (2.8333, 27.9557)
  arc A284 (16.3333, 47.5057) -> (16.8333, 47.0057) centre (16.3333, 47.0057) cw
  line L284 (2.8333, 34.0057) -> (2.8333, 47.0057)
  line L285 (3.3333, 47.5057) -> (16.3333, 47.5057)
  arc A285 (16.8333, 34.0057) -> (16.3333, 33.5057) centre (16.3333, 34.0057) cw
  line L286 (16.8333, 47.0057) -> (16.8333, 34.0057)
  line L287 (16.3333, 33.5057) -> (3.3333, 33.5057)
  arc A286 (2.8333, 47.0057) -> (3.3333, 47.5057) centre (3.3333, 47.0057) cw
  arc A287 (3.3333, 33.5057) -> (2.8333, 34.0057) centre (3.3333, 34.0057) cw
  line L288 (16.3333, 52.5557) -> (3.3333, 52.5557)
  arc A288 (16.8333, 53.0557) -> (16.3333, 52.5557) centre (16.3333, 53.0557) cw
  line L289 (2.8333, 53.0557) -> (2.8333, 66.0557)
  arc A289 (3.3333, 52.5557) -> (2.8333, 53.0557) centre (3.3333, 53.0557) cw
  line L290 (3.3333, 66.5557) -> (16.3333, 66.5557)
  line L291 (16.8333, 66.0557) -> (16.8333, 53.0557)
  arc A290 (16.3333, 66.5557) -> (16.8333, 66.0557) centre (16.3333, 66.0557) cw
  arc A291 (2.8333, 66.0557) -> (3.3333, 66.5557) centre (3.3333, 66.0557) cw
  arc A292 (2.8333, 85.1057) -> (3.3333, 85.6057) centre (3.3333, 85.1057) cw
  line L292 (3.3333, 85.6057) -> (16.3333, 85.6057)
  arc A293 (3.3333, 71.6057) -> (2.8333, 72.1057) centre (3.3333, 72.1057) cw
  arc A294 (16.8333, 72.1057) -> (16.3333, 71.6057) centre (16.3333, 72.1057) cw
  line L293 (2.8333, 72.1057) -> (2.8333, 85.1057)
  line L294 (16.3333, 71.6057) -> (3.3333, 71.6057)
  arc A295 (16.3333, 85.6057) -> (16.8333, 85.1057) centre (16.3333, 85.1057) cw
  line L295 (16.8333, 85.1057) -> (16.8333, 72.1057)
  line L296 (16.3333, 90.6557) -> (3.3333, 90.6557)
  arc A296 (2.8333, 104.1557) -> (3.3333, 104.6557) centre (3.3333, 104.1557) cw
  line L297 (3.3333, 104.6557) -> (16.3333, 104.6557)
  arc A297 (3.3333, 90.6557) -> (2.8333, 91.1557) centre (3.3333, 91.1557) cw
  arc A298 (16.8333, 91.1557) -> (16.3333, 90.6557) centre (16.3333, 91.1557) cw
  arc A299 (16.3333, 104.6557) -> (16.8333, 104.1557) centre (16.3333, 104.1557) cw
  line L298 (2.8333, 91.1557) -> (2.8333, 104.1557)
  line L299 (16.8333, 104.1557) -> (16.8333, 91.1557)
  arc A300 (16.8333, 110.2057) -> (16.3333, 109.7057) centre (16.3333, 110.2057) cw
  line L300 (16.8333, 123.2057) -> (16.8333, 110.2057)
  arc A301 (3.3333, 109.7057) -> (2.8333, 110.2057) centre (3.3333, 110.2057) cw
  line L301 (16.3333, 109.7057) -> (3.3333, 109.7057)
  arc A302 (16.3333, 123.7057) -> (16.8333, 123.2057) centre (16.3333, 123.2057) cw
  line L302 (2.8333, 110.2057) -> (2.8333, 123.2057)
  line L303 (3.3333, 123.7057) -> (16.3333, 123.7057)
  arc A303 (2.8333, 123.2057) -> (3.3333, 123.7057) centre (3.3333, 123.2057) cw
  arc A304 (22.3832, -214.1443) -> (21.8833, -213.6443) centre (22.3832, -213.6443) cw
  line L304 (35.3833, -214.1443) -> (22.3832, -214.1443)
  arc A305 (35.8833, -213.6443) -> (35.3833, -214.1443) centre (35.3832, -213.6443) cw
  arc A306 (21.8832, -200.6443) -> (22.3833, -200.1443) centre (22.3833, -200.6443) cw
  line L305 (35.8833, -200.6443) -> (35.8833, -213.6443)
  line L306 (21.8833, -213.6443) -> (21.8832, -200.6443)
  arc A307 (35.3833, -200.1443) -> (35.8833, -200.6443) centre (35.3833, -200.6443) cw
  line L307 (22.3833, -200.1443) -> (35.3833, -200.1443)
  arc A308 (35.3833, -181.0943) -> (35.8833, -181.5943) centre (35.3833, -181.5943) cw
  arc A309 (35.8833, -194.5943) -> (35.3833, -195.0943) centre (35.3833, -194.5943) cw
  line L308 (22.3833, -181.0943) -> (35.3833, -181.0943)
  line L309 (35.3833, -195.0943) -> (22.3833, -195.0943)
  arc A310 (21.8833, -181.5943) -> (22.3833, -181.0943) centre (22.3833, -181.5943) cw
  line L310 (35.8833, -181.5943) -> (35.8833, -194.5943)
  line L311 (21.8833, -194.5943) -> (21.8833, -181.5943)
  arc A311 (22.3833, -195.0943) -> (21.8833, -194.5943) centre (22.3833, -194.5943) cw
  arc A312 (21.8833, -162.5443) -> (22.3833, -162.0443) centre (22.3833, -162.5443) cw
  line L312 (35.8833, -162.5443) -> (35.8833, -175.5443)
  line L313 (22.3833, -162.0443) -> (35.3833, -162.0443)
  line L314 (21.8833, -175.5443) -> (21.8833, -162.5443)
  arc A313 (35.3833, -162.0443) -> (35.8833, -162.5443) centre (35.3833, -162.5443) cw
  line L315 (35.3833, -176.0443) -> (22.3833, -176.0443)
  arc A314 (35.8833, -175.5443) -> (35.3833, -176.0443) centre (35.3833, -175.5443) cw
  arc A315 (22.3833, -176.0443) -> (21.8833, -175.5443) centre (22.3833, -175.5443) cw
  line L316 (31.4083, -156.4943) -> (31.4083, -143.4943)
  line L317 (45.4083, -143.4943) -> (45.4083, -156.4943)
  line L318 (31.9083, -142.9943) -> (44.9083, -142.9943)
  arc A316 (31.9083, -156.9943) -> (31.4083, -156.4943) centre (31.9083, -156.4943) cw
  arc A317 (31.4083, -143.4943) -> (31.9083, -142.9943) centre (31.9083, -143.4943) cw
  arc A318 (45.4083, -156.4943) -> (44.9083, -156.9943) centre (44.9082, -156.4943) cw
  arc A319 (44.9083, -142.9943) -> (45.4083, -143.4943) centre (44.9083, -143.4943) cw
  line L319 (44.9083, -156.9943) -> (31.9083, -156.9943)
  arc A320 (23.4703, -155.9943) -> (22.9703, -155.4943) centre (23.4703, -155.4943) cw
  arc A321 (29.4703, -140.9943) -> (29.9703, -141.4943) centre (29.4703, -141.4943) cw
  line L320 (29.4703, -155.9943) -> (23.4703, -155.9943)
  line L321 (29.9703, -141.4943) -> (29.9703, -155.4943)
  line L322 (23.4703, -140.9943) -> (29.4703, -140.9943)
  arc A322 (29.9703, -155.4943) -> (29.4703, -155.9943) centre (29.4702, -155.4943) cw
  line L323 (22.9703, -155.4943) -> (22.9703, -141.4943)
  arc A323 (22.9703, -141.4943) -> (23.4703, -140.9943) centre (23.4703, -141.4943) cw
  arc A324 (53.3463, -140.9943) -> (53.8463, -141.4943) centre (53.3463, -141.4943) cw
  line L324 (53.3463, -155.9943) -> (47.3463, -155.9943)
  arc A325 (47.3463, -155.9943) -> (46.8463, -155.4943) centre (47.3463, -155.4943) cw
  line L325 (46.8463, -155.4943) -> (46.8463, -141.4943)
  arc A326 (53.8462, -155.4943) -> (53.3463, -155.9943) centre (53.3463, -155.4943) cw
  line L326 (47.3463, -140.9943) -> (53.3463, -140.9943)
  line L327 (53.8463, -141.4943) -> (53.8462, -155.4943)
  arc A327 (46.8463, -141.4943) -> (47.3463, -140.9943) centre (47.3463, -141.4943) cw
  line L328 (35.3833, -118.8943) -> (22.3833, -118.8943)
  arc A328 (22.3833, -118.8943) -> (21.8833, -118.3943) centre (22.3833, -118.3943) cw
  line L329 (21.8833, -118.3943) -> (21.8833, -105.3943)
  line L330 (22.3833, -104.8943) -> (35.3833, -104.8943)
  arc A329 (35.8833, -118.3943) -> (35.3833, -118.8943) centre (35.3833, -118.3943) cw
  arc A330 (21.8833, -105.3943) -> (22.3833, -104.8943) centre (22.3833, -105.3943) cw
  arc A331 (35.3833, -104.8943) -> (35.8833, -105.3943) centre (35.3833, -105.3943) cw
  line L331 (35.8833, -105.3943) -> (35.8833, -118.3943)
  line L332 (22.8833, -126.8323) -> (22.8833, -120.8323)
  line L333 (37.3833, -127.3323) -> (23.3833, -127.3323)
  line L334 (23.3833, -120.3323) -> (37.3833, -120.3323)
  arc A332 (23.3833, -127.3323) -> (22.8833, -126.8323) centre (23.3833, -126.8323) cw
  line L335 (37.8833, -120.8323) -> (37.8833, -126.8323)
  arc A333 (22.8833, -120.8323) -> (23.3833, -120.3323) centre (23.3833, -120.8323) cw
  arc A334 (37.3833, -120.3323) -> (37.8833, -120.8323) centre (37.3833, -120.8323) cw
  arc A335 (37.8833, -126.8323) -> (37.3833, -127.3323) centre (37.3833, -126.8323) cw
  arc A336 (37.3833, -96.4563) -> (37.8833, -96.9563) centre (37.3833, -96.9563) cw
  arc A337 (23.3833, -103.4563) -> (22.8833, -102.9563) centre (23.3833, -102.9563) cw
  line L336 (37.8833, -96.9563) -> (37.8833, -102.9563)
  arc A338 (22.8833, -96.9563) -> (23.3833, -96.4563) centre (23.3833, -96.9563) cw
  line L337 (22.8833, -102.9563) -> (22.8833, -96.9563)
  line L338 (23.3833, -96.4563) -> (37.3833, -96.4563)
  arc A339 (37.8833, -102.9563) -> (37.3833, -103.4563) centre (37.3833, -102.9563) cw
  line L339 (37.3833, -103.4563) -> (23.3833, -103.4563)
  line L340 (35.8833, -76.8193) -> (35.8833, -89.8193)
  arc A340 (35.8833, -89.8193) -> (35.3833, -90.3193) centre (35.3833, -89.8193) cw
  arc A341 (22.3833, -90.3193) -> (21.8833, -89.8193) centre (22.3833, -89.8193) cw
  line L341 (22.3833, -76.3193) -> (35.3833, -76.3193)
  arc A342 (21.8833, -76.8193) -> (22.3833, -76.3193) centre (22.3833, -76.8193) cw
  line L342 (21.8833, -89.8193) -> (21.8833, -76.8193)
  line L343 (35.3833, -90.3193) -> (22.3833, -90.3193)
  arc A343 (35.3833, -76.3193) -> (35.8833, -76.8193) centre (35.3833, -76.8193) cw
  line L344 (35.3833, -71.2693) -> (22.3833, -71.2693)
  line L345 (22.3833, -57.2693) -> (35.3833, -57.2693)
  arc A344 (21.8833, -57.7693) -> (22.3833, -57.2693) centre (22.3833, -57.7693) cw
  arc A345 (35.3833, -57.2693) -> (35.8833, -57.7693) centre (35.3833, -57.7693) cw
  line L346 (35.8833, -57.7693) -> (35.8833, -70.7693)
  arc A346 (35.8833, -70.7693) -> (35.3833, -71.2693) centre (35.3833, -70.7693) cw
  arc A347 (22.3833, -71.2693) -> (21.8833, -70.7693) centre (22.3833, -70.7693) cw
  line L347 (21.8833, -70.7693) -> (21.8833, -57.7693)
  arc A348 (22.3833, -52.2193) -> (21.8833, -51.7193) centre (22.3833, -51.7193) cw
  line L348 (21.8833, -51.7193) -> (21.8833, -38.7193)
  line L349 (22.3833, -38.2193) -> (35.3833, -38.2193)
  arc A349 (35.8833, -51.7193) -> (35.3833, -52.2193) centre (35.3833, -51.7193) cw
  arc A350 (21.8833, -38.7193) -> (22.3833, -38.2193) centre (22.3833, -38.7193) cw
  line L350 (35.8833, -38.7193) -> (35.8833, -51.7193)
  arc A351 (35.3833, -38.2193) -> (35.8833, -38.7193) centre (35.3833, -38.7193) cw
  line L351 (35.3833, -52.2193) -> (22.3833, -52.2193)
  arc A352 (35.8833, -32.6693) -> (35.3833, -33.1693) centre (35.3833, -32.6693) cw
  line L352 (35.8833, -19.6693) -> (35.8833, -32.6693)
  line L353 (22.3833, -19.1693) -> (35.3833, -19.1693)
  line L354 (35.3833, -33.1693) -> (22.3833, -33.1693)
  arc A353 (21.8833, -19.6693) -> (22.3833, -19.1693) centre (22.3833, -19.6693) cw